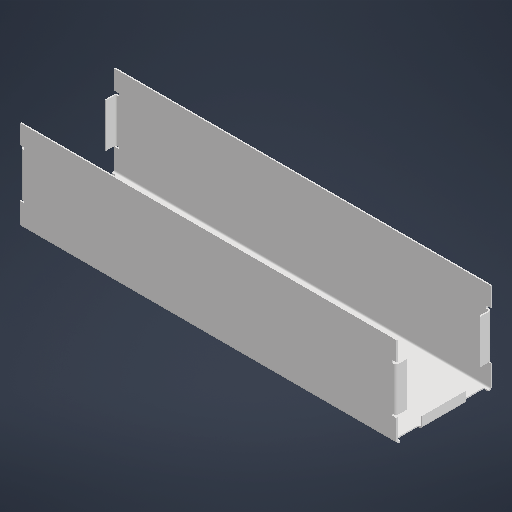
# Autodesk Inventor part: Bottom
Saved by Autodesk Inventor 2026.1 (Build 301233020, 233B)
## iProperties
Created: 2025-11-02
Part Number: Bottom
Material: Generic
Document SubType Name: Sheet Metal
Designer: 박정현
Density: 1 g/cm^3
Sheet Metal Rule: Default
Appearance: Default
Author: 박정현
Autodesk Inventor part; units mm, degrees
ref_plane "YZ Plane" through (0, 0, 0) normal (1, 0, 0) x (0, 1, 0)
ref_plane "XZ Plane" through (0, 0, 0) normal (0, 1, 0) x (-1, 0, 0)
ref_plane "XY Plane" through (0, 0, 0) normal (0, 0, 1) x (1, 0, 0)
sketch "Sketch1" plane through (0, 0, 0) normal (0, 1, 0) x (-1, 0, 0)
  line L0 (210, -50) -> (-210, -50)
  line L1 (-210, -50) -> (-210, 50)
  line L2 (-210, 50) -> (210, 50)
  line L3 (210, 50) -> (210, -50)
  line L4 (215, 50) -> (-215, 50)
  line L5 (-215, 50) -> (-215, 78)
  line L6 (-215, 78) -> (215, 78)
  line L7 (215, 78) -> (215, 50)
  line L8 (215, -50) -> (-215, -50)
  line L9 (-215, -50) -> (-215, -78)
  line L10 (-215, -78) -> (215, -78)
  line L11 (215, -78) -> (215, -50)
  line L12 (210, 78) -> (-210, 78)
  line L13 (-210, 78) -> (-210, 133)
  line L14 (-210, 133) -> (210, 133)
  line L15 (210, 133) -> (210, 78)
  line L16 (215, 133) -> (-215, 133)
  line L17 (-215, 133) -> (-215, 155)
  line L18 (-215, 155) -> (215, 155)
  line L19 (215, 155) -> (215, 133)
  line L20 (210, -78) -> (-210, -78)
  line L21 (-210, -78) -> (-210, -133)
  line L22 (-210, -133) -> (210, -133)
  line L23 (210, -133) -> (210, -78)
  line L24 (215, -133) -> (-215, -133)
  line L25 (-215, -133) -> (-215, -155)
  line L26 (-215, -155) -> (215, -155)
  line L27 (215, -155) -> (215, -133)
  line L28 (210, -25) -> (215, -25)
  line L29 (215, -25) -> (215, 25)
  line L30 (215, 25) -> (210, 25)
  line L31 (210, 25) -> (210, -25)
  line L32 (215, -25) -> (225, -25)
  line L33 (225, -25) -> (225, 25)
  line L34 (225, 25) -> (215, 25)
  line L35 (215, 25) -> (215, -25)
  line L36 (-210, -25) -> (-215, -25)
  line L37 (-215, -25) -> (-215, 25)
  line L38 (-215, 25) -> (-210, 25)
  line L39 (-210, 25) -> (-210, -25)
  line L40 (-215, -25) -> (-225, -25)
  line L41 (-225, -25) -> (-225, 25)
  line L42 (-225, 25) -> (-215, 25)
  line L43 (-215, 25) -> (-215, -25)
  line L44 (210, 80) -> (215, 80)
  line L45 (215, 80) -> (215, 130)
  line L46 (215, 130) -> (210, 130)
  line L47 (210, 130) -> (210, 80)
  line L48 (215, 80) -> (225, 80)
  line L49 (225, 80) -> (225, 130)
  line L50 (225, 130) -> (215, 130)
  line L51 (215, 130) -> (215, 80)
  line L52 (-210, 80) -> (-215, 80)
  line L53 (-215, 80) -> (-215, 130)
  line L54 (-215, 130) -> (-210, 130)
  line L55 (-210, 130) -> (-210, 80)
  line L56 (-215, 80) -> (-225, 80)
  line L57 (-225, 80) -> (-225, 130)
  line L58 (-225, 130) -> (-215, 130)
  line L59 (-215, 130) -> (-215, 80)
  line L60 (210, -130) -> (215, -130)
  line L61 (215, -130) -> (215, -80)
  line L62 (215, -80) -> (210, -80)
  line L63 (210, -80) -> (210, -130)
  line L64 (215, -130) -> (225, -130)
  line L65 (225, -130) -> (225, -80)
  line L66 (225, -80) -> (215, -80)
  line L67 (215, -80) -> (215, -130)
  line L68 (-210, -130) -> (-215, -130)
  line L69 (-215, -130) -> (-215, -80)
  line L70 (-215, -80) -> (-210, -80)
  line L71 (-210, -80) -> (-210, -130)
  line L72 (-215, -130) -> (-225, -130)
  line L73 (-225, -130) -> (-225, -80)
  line L74 (-225, -80) -> (-215, -80)
  line L75 (-215, -80) -> (-215, -130)
  line L76 (210, 50) -> (-210, -50) construction
  line L77 (-210, 50) -> (210, -50) construction
  line L78 (215, -55) -> (-215, -55) construction
  line L79 (215, 55) -> (-215, 55) construction
  point P0 (0, 0)
  point P1 (210, 0)
  point P2 (-210, 0)
  point P3 (210, 50)
  point P4 (-210, 133)
  point P5 (-210, 78)
  point P6 (-210, -50)
  point P7 (-210, -78)
  point P8 (-210, -133)
  dimension "d0" = 430
  dimension "d1" = 5
  dimension "d2" = 5
  dimension "d3" = 100
  dimension "d4" = 50
  dimension "d5" = 50
  dimension "d6" = 5
  dimension "d7" = 5
  dimension "d8" = 50
  dimension "d9" = 50
  dimension "d10" = 10
  dimension "d11" = 10
  dimension "d12" = 105
  dimension "d13" = 105
  dimension "d14" = 28
  dimension "d15" = 28
  dimension "d16" = 25
  dimension "d17" = 25
  dimension "d18" = 22
  dimension "d19" = 22
  dimension "d57" = 5
  dimension "d58" = 5
  constraints: 160 end point, 39 point on line, 38 parallel, 21 perpendicular, 19 horizontal, 6 midpoint, 5 collinear, 1 other
  measures "d0" distance of L17.end L18.end
  measures "d1" distance between parallel lines of L15 L19
  measures "d2" distance between parallel lines of L13 L17
  measures "d3" distance between parallel lines of L0 L2
  measures "d4" distance of L32.end L33.end
  measures "d5" distance of L40.end L41.end
  measures "d6" distance of L45.end L46.end
  measures "d7" distance between parallel lines of L13 L53
  measures "d8" distance of L48.end L49.end
  measures "d9" distance of L64.end L65.end
  measures "d10" distance of L33.end L34.end
  measures "d11" distance of L41.end L42.end
  measures "d12" distance between parallel lines of L4 L18
  measures "d13" distance between parallel lines of L26 L8
  measures "d14" distance between parallel lines of L8 L10
  measures "d15" distance between parallel lines of L4 L6
  measures "d16" distance between parallel lines of L64 L26
  measures "d17" distance between parallel lines of L50 L18
  measures "d18" distance between parallel lines of L18 L16
  measures "d19" distance between parallel lines of L26 L24
  measures "d57" distance between parallel lines of L8 L78
  measures "d58" distance between parallel lines of L2 L79
extrude "Plate1" add sketch "Sketch1" against normal blind 1.5
fold "Fold1" angle 90 bend radius 1.5 thickness 1.5 k factor 0.44 line from (-215, 0, -80) to (-215, 0, -130) line at bend end moving side (-1, 0, 0) folds toward (0, 1, 0)
fold "Fold2" angle 90 bend radius 1.5 thickness 1.5 k factor 0.44 line from (-215, 0, -25) to (-215, 0, 25) line at bend end moving side (-1, 0, 0) folds toward (0, 1, 0)
fold "Fold3" angle 90 bend radius 1.5 thickness 1.5 k factor 0.44 line from (-215, 0, 130) to (-215, 0, 80) line at bend end moving side (-1, 0, 0) folds toward (0, 1, 0)
fold "Fold4" angle 90 bend radius 1.5 thickness 1.5 k factor 0.44 line from (215, 0, -80) to (215, 0, -130) line at bend end moving side (1, 0, 0) folds toward (0, 1, 0)
fold "Fold5" angle 90 bend radius 1.5 thickness 1.5 k factor 0.44 line from (215, 0, 25) to (215, 0, -25) line at bend end moving side (1, 0, 0) folds toward (0, 1, 0)
fold "Fold6" angle 90 bend radius 1.5 thickness 1.5 k factor 0.44 line from (215, 0, 80) to (215, 0, 130) line at bend end moving side (1, 0, 0) folds toward (0, 1, 0)
fold "Fold7" angle 90 bend radius 1.5 thickness 1.5 k factor 0.44 line from (-215, 0, -55) to (215, 0, -55) line at bend end moving side (0, 0, -1) folds toward (0, 1, 0)
fold "Fold8" angle 90 bend radius 1.5 thickness 1.5 k factor 0.44 line from (-215, 0, 55) to (215, 0, 55) line at bend end moving side (0, 0, 1) folds toward (0, 1, 0)
equation "\"d2\" = d1"
equation "\"d5\" = d4"
equation "\"d6\" = d1"
equation "\"d7\" = d1"
equation "\"d8\" = d4"
equation "\"d9\" = d4"
equation "\"d11\" = d10"
equation "\"BendRadius\" = Thickness"
equation "\"BendReliefWidth\" = Thickness"
equation "\"BendReliefDepth\" = 0.5 * Thickness"
equation "\"CornerReliefSize\" = 4 * Thickness"
equation "\"MinimumRemnant\" = 2 * Thickness"
equation "\"TransitionRadius\" = BendRadius"
equation "\"JacobiRadiusSize\" = BendRadius"
equation "\"GapSize\" = Thickness"
equation "\"Thickness\" = 1.5"
body "Solid1"
